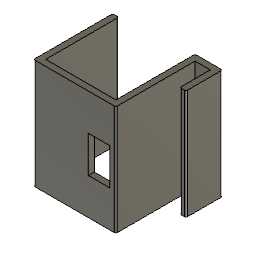
mmWave Sensor MacBook Pro Hook (Autodesk Fusion 360 design; units mm, degrees)
part number: 2026-05-11-10-35-28-776
Autodesk Fusion 360 part; units mm, degrees
sketch "Sketch2" plane through (0, 0, 0) normal (0, 0, 1) x (1, 0, 0)
  line L0 (0, 0) -> (2, 0)
  line L1 (2, 0) -> (2, 10)
  line L2 (2, 10) -> (0, 10)
  line L3 (0, 10) -> (0, 0)
  line L4 (0, 10) -> (2, 10)
  line L5 (2, 10) -> (2, 12)
  line L6 (2, 12) -> (0, 12)
  line L7 (0, 12) -> (0, 10)
  line L8 (0, 10) -> (-5, 10)
  line L9 (-5, 10) -> (-5, 12)
  line L10 (-5, 12) -> (0, 12)
  line L11 (0, 12) -> (0, 10)
  line L12 (-5, 10) -> (-7, 10)
  line L13 (-7, 10) -> (-7, 12)
  line L14 (-7, 12) -> (-5, 12)
  line L15 (-5, 12) -> (-5, 10)
  line L16 (-7, 10) -> (-5, 10)
  line L17 (-5, 10) -> (-5, -14)
  line L18 (-5, -14) -> (-7, -14)
  line L19 (-7, -14) -> (-7, 10)
  line L20 (-7, -14) -> (-5, -14)
  line L21 (-5, -14) -> (-5, -16)
  line L22 (-5, -16) -> (-7, -16)
  line L23 (-7, -16) -> (-7, -14)
  line L24 (-7, -16) -> (-30, -16)
  line L25 (-30, -16) -> (-30, -14)
  line L26 (-30, -14) -> (-7, -14)
  line L27 (-7, -14) -> (-7, -16)
  line L28 (-30, -16) -> (-32, -16)
  line L29 (-32, -16) -> (-32, -14)
  line L30 (-32, -14) -> (-30, -14)
  line L31 (-30, -14) -> (-30, -16)
  line L32 (-32, -14) -> (-30, -14)
  line L33 (-30, -14) -> (-30, 10)
  line L34 (-30, 10) -> (-32, 10)
  line L35 (-32, 10) -> (-32, -14)
  dimension "d3" = 2
  dimension "d4" = 10
  dimension "d5" = 2
  dimension "d6" = 2
  dimension "d7" = 5
  dimension "d8" = 2
  dimension "d9" = 2
  dimension "d10" = 2
  dimension "d11" = 24
  dimension "d12" = 2
  dimension "d13" = 23
  dimension "d14" = 2
  dimension "d15" = 2
  dimension "d16" = 2
  dimension "d17" = 2
  dimension "d18" = 24
  constraint horizontal L0
  constraint vertical L1
  constraint horizontal L2
  constraint vertical L3
  constraint coincident L0.start L3.end
  constraint horizontal L4
  constraint vertical L5
  constraint horizontal L6
  constraint vertical L7
  constraint horizontal L8
  constraint vertical L9
  constraint horizontal L10
  constraint vertical L11
  constraint horizontal L12
  constraint vertical L13
  constraint horizontal L14
  constraint vertical L15
  constraint horizontal L16
  constraint vertical L17
  constraint horizontal L18
  constraint vertical L19
  constraint horizontal L20
  constraint vertical L21
  constraint horizontal L22
  constraint vertical L23
  constraint horizontal L24
  constraint vertical L25
  constraint horizontal L26
  constraint vertical L27
  constraint horizontal L28
  constraint vertical L29
  constraint horizontal L30
  constraint vertical L31
  constraint horizontal L32
  constraint vertical L33
  constraint horizontal L34
  constraint vertical L35
  measures "d3" distance of L0.start L0.end
  measures "d4" distance of L0.start L2.end
  measures "d5" distance of L2.end L1.end
  measures "d6" distance of L2.end L6.end
  measures "d7" distance of L2.end L8.end
  measures "d8" distance of L2.end L6.end
  measures "d9" distance of L8.end L12.end
  measures "d10" distance of L8.end L9.end
  measures "d11" distance of L12.end L18.end
  measures "d12" distance of L18.end L22.end
  measures "d13" distance of L22.end L24.end
  measures "d14" distance of L22.end L18.end
  measures "d15" distance of L24.end L28.end
  measures "d16" distance of L24.end L25.end
  measures "d17" distance of L29.end L25.end
  measures "d18" distance of L29.end L34.end
extrude "Extrude1" add sketch "Sketch2" along normal blind 36
sketch "Sketch3" plane through (0, -16, 0) normal (0, -1, 0) x (1, 0, 0)
  line L0 (-32, 0) -> (-5, 0)
  line L1 (-5, 0) -> (-5, 36)
  line L2 (-5, 36) -> (-32, 36)
  line L3 (-32, 36) -> (-32, 0)
  line L4 (-5, 18) -> (-7, 18) construction
  line L5 (-7, 18) -> (-10.5, 18) construction
  line L6 (-14, 12) -> (-7, 12)
  line L7 (-7, 12) -> (-7, 24)
  line L8 (-7, 24) -> (-14, 24)
  line L9 (-14, 24) -> (-14, 12)
  line L10 (-14, 12) -> (-7, 24) construction
  line L11 (-7, 12) -> (-14, 24) construction
  point P0 (-7, 18)
  point P1 (-10.5, 18)
  dimension "d23" = 2
  dimension "d28" = 3.5
  dimension "d29" = 7
  dimension "d30" = 12
  constraint midpoint L1 L4.start
  constraint perpendicular L1 L4
  constraint coincident P0 L4.end
  constraint horizontal L5
  constraint horizontal L6
  constraint perpendicular L6 L7
  constraint parallel L6 L8
  constraint parallel L7 L9
  constraint coincident L10 P1
  constraint coincident L11 P1
  constraint coincident P1 L5.end
  measures "d23" distance of L4.start P0
  measures "d28" distance of P0 P1
  measures "d29" distance of L7.end L8.end
  measures "d30" distance of L6.end L7.end
extrude "Extrude3" cut sketch "Sketch3" against normal blind 3 contours L6 L7 L8 L9
fillet "Fillet1" radius 0.5 8 edges at (0, 0, 18) (2, 0, 18) (-5, -16, 18) (-32, -16, 18) (2, 12, 18) (-7, 12, 18) (-30, 10, 18) (-32, 10, 18)
